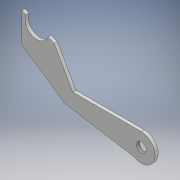
# Autodesk Inventor part: efektor szczypce1
Saved by Autodesk Inventor 2017.3 (Build 213256000, 256)
## iProperties
Created: 2019-03-17
Part Number: efektor szczypce1
Material: Ogólny
Document SubType Name: Modeling
Designer: legox
Density: 1 g/cm^3
Appearance: Domyślna
Author: legox
Autodesk Inventor part; units mm, degrees
ref_plane "YZ Plane" through (0, 0, 0) normal (1, 0, 0) x (0, 1, 0)
ref_plane "XZ Plane" through (0, 0, 0) normal (0, 1, 0) x (-1, 0, 0)
ref_plane "XY Plane" through (0, 0, 0) normal (0, 0, 1) x (1, 0, 0)
sketch "Szkic1" plane through (0, 0, 0) normal (0, 1, 0) x (-1, 0, 0)
  arc A0 (0, 7) -> (3.6056, -6) centre (0, 0) ccw
  line L0 (3.6056, -6) -> (39.2808, 0)
  line L1 (44.4792, 23.7708) -> (35, 7)
  line L2 (35, 7) -> (0, 7)
  circle A1 centre (0, 0) radius 2.5
  line L3 (61, 30) -> (61, 15)
  line L4 (61, 15) -> (39.2808, 0)
  arc A2 (47.6958, 24.9837) -> (58.9242, 29.2173) centre (53.31, 27.1005) ccw
  line L5 (44.4792, 23.7708) -> (47.6958, 24.9837)
  line L6 (58.9242, 29.2173) -> (61, 30)
  dimension "d0" = 14
  dimension "d1" = 5
  dimension "d5" = 12
  constraints: 14 end point, 4 point on circle, 3 centre point, 2 coincident, 1 vertical
  measures "d0" diameter of A0
  measures "d1" diameter of A1
  measures "d5" diameter of A2
extrude "Wyciągnięcie proste1" add sketch "Szkic1" along normal blind 1.6
